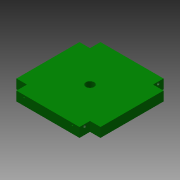
# Autodesk Inventor part: PEEKplate
Saved by Autodesk Inventor 2015 SP1 (Build 190203100, 203)
## iProperties
Created: 2015-09-28
Part Number: PEEKplate
Material: Generic
Document SubType Name: Modeling
Designer: I Rabey
Density: 1 g/cm^3
Appearance: Default
Author: I Rabey
Autodesk Inventor part; units mm, degrees
ref_plane "YZ Plane" through (0, 0, 0) normal (1, 0, 0) x (0, 1, 0)
ref_plane "XZ Plane" through (0, 0, 0) normal (0, 1, 0) x (-1, 0, 0)
ref_plane "XY Plane" through (0, 0, 0) normal (0, 0, 1) x (1, 0, 0)
sketch "Sketch1" plane through (0, 0, 0) normal (0, 1, 0) x (-1, 0, 0)
  line L0 (51.3, 38.5) -> (51.3, -38.5)
  line L1 (51.3, -38.5) -> (38.5, -38.5)
  line L2 (38.5, -38.5) -> (38.5, -51.3)
  line L3 (38.5, -51.3) -> (-38.5, -51.3)
  line L4 (-38.5, -51.3) -> (-38.5, -38.5)
  line L5 (-38.5, -38.5) -> (-51.3, -38.5)
  line L6 (-51.3, -38.5) -> (-51.3, 38.5)
  line L7 (-51.3, 38.5) -> (-38.5, 38.5)
  line L8 (-38.5, 38.5) -> (-38.5, 51.3)
  line L9 (-38.5, 51.3) -> (38.5, 51.3)
  line L10 (38.5, 51.3) -> (38.5, 38.5)
  line L11 (38.5, 38.5) -> (51.3, 38.5)
  circle A0 centre (0, 0) radius 5
  dimension "d0" = 77
  dimension "d1" = 12.8
  dimension "d2" = 12.8
  dimension "d3" = 77
  dimension "d4" = 12.8
  dimension "d5" = 12.8
  dimension "d6" = 77
  dimension "d7" = 12.8
  dimension "d8" = 12.8
  dimension "d9" = 77
  dimension "d10" = 12.8
  dimension "d11" = 12.8
  dimension "d12" = 38.5
  dimension "d13" = 51.3
  dimension "d14" = 10
  constraints: 24 end point, 7 point on line, 3 perpendicular, 1 centre point, 1 coincident, 1 horizontal, 1 vertical
  measures "d0" distance of L0.start L0.end
  measures "d1" distance of L0.end L1.end
  measures "d2" distance of L1.end L2.end
  measures "d3" distance of L2.end L3.end
  measures "d4" distance of L3.end L4.end
  measures "d5" distance of L4.end L5.end
  measures "d6" distance of L5.end L6.end
  measures "d7" distance of L6.end L7.end
  measures "d8" distance of L7.end L8.end
  measures "d9" distance of L8.end L9.end
  measures "d10" distance of L9.end L10.end
  measures "d11" distance of L10.end L11.end
  measures "d12" distance from line of L1 point (0, 0)
  measures "d13" distance from line of L0 point (0, 0)
  measures "d14" diameter of A0
extrude "Extrusion1" add sketch "Sketch1" along normal blind 11.5
sketch "Sketch2" plane through (38.5, 0, 51.3) normal (1, 0, 0) x (0, 0, -1)
  circle A0 centre (6.4, 9) radius 1.65
  line L0 (0, 0) -> (0, 11.5) projected
  line L1 (0, 11.5) -> (12.8, 11.5) projected
  point P0 (51.3, 0)
  dimension "d17" = 3.3
  dimension "d18" = 6.4
  dimension "d19" = 2.5
  constraints: 1 centre point
  measures "d17" diameter of A0
  measures "d18" distance from line of A0.centre L0
  measures "d19" distance from line of L1 A0.centre
hole "Hole1" at (38.5, 9, 44.9) direction (-1, 0, 0) diameter 3.3 depth 10 tip angle 118
thread "Thread1" size "M3.5x0.6" class "6H" standard "ANSI Metric M Profile" full length
sketch "Sketch3" plane through (-38.5, 0, 51.3) normal (0, 0, 1) x (1, 0, 0)
  circle A0 centre (68, 9) radius 0.5
  line L0 (0, 11.5) -> (77, 11.5) projected
  line L1 (77, 0) -> (77, 11.5) projected
  point P0 (38.5, 0)
  dimension "d29" = 1
  dimension "d30" = 2.5
  dimension "d31" = 9
  constraints: 1 centre point
  measures "d29" diameter of A0
  measures "d30" distance from line of L0 A0.centre
  measures "d31" distance from line of A0.centre L1
hole "Hole2" at (29.5, 9, 51.3) direction (0, 0, -1) diameter 2 depth 5 tip angle 118
sketch "Sketch4" plane through (-38.5, 0, 38.5) normal (-1, 0, 0) x (0, 0, 1)
  circle A0 centre (6.4, 9) radius 1.65
  line L0 (0, 11.5) -> (12.8, 11.5) projected
  line L1 (12.8, 0) -> (12.8, 11.5) projected
  point P0 (-38.5, 0)
  dimension "d39" = 3.3
  dimension "d40" = 2.5
  dimension "d41" = 6.4
  constraints: 1 centre point
  measures "d39" diameter of A0
  measures "d40" distance from line of L0 A0.centre
  measures "d41" distance from line of L1 A0.centre
hole "Hole3" at (-38.5, 9, 44.9) direction (1, 0, 0) diameter 3.3 depth 10 tip angle 118
thread "Thread2" size "M3.5x0.6" class "6H" standard "ANSI Metric M Profile" full length
sketch "Sketch5" plane through (-38.5, 0, 51.3) normal (0, 0, 1) x (1, 0, 0)
  circle A0 centre (9, 9) radius 1
  line L0 (0, 0) -> (0, 11.5) projected
  line L1 (0, 11.5) -> (77, 11.5) projected
  point P0 (38.5, 0)
  dimension "d51" = 2
  dimension "d52" = 9
  dimension "d53" = 2.5
  constraints: 1 centre point
  measures "d51" diameter of A0
  measures "d52" distance from line of A0.centre L0
  measures "d53" distance from line of L1 A0.centre
hole "Hole4" at (-29.5, 9, 51.3) direction (0, 0, -1) diameter 2 depth 5 tip angle 118
sketch "Sketch6" plane through (38.5, 0, -38.5) normal (1, 0, 0) x (0, 0, -1)
  circle A0 centre (6.4, 9) radius 1.65
  line L0 (0, 11.5) -> (12.8, 11.5) projected
  line L1 (12.8, 0) -> (12.8, 11.5) projected
  point P0 (-38.5, 0)
  dimension "d61" = 3.3
  dimension "d62" = 2.5
  dimension "d63" = 6.4
  constraints: 1 centre point
  measures "d61" diameter of A0
  measures "d62" distance from line of A0.centre L0
  measures "d63" distance from line of L1 A0.centre
hole "Hole5" at (38.5, 9, -44.9) direction (-1, 0, 0) diameter 3.3 depth 10 tip angle 118
thread "Thread3" size "M3.5x0.6" class "6H" standard "ANSI Metric M Profile" full length
sketch "Sketch7" plane through (38.5, 0, -51.3) normal (0, 0, -1) x (-1, 0, 0)
  circle A0 centre (9, 9) radius 1
  line L0 (0, 0) -> (0, 11.5) projected
  line L1 (0, 11.5) -> (77, 11.5) projected
  point P0 (38.5, 0)
  dimension "d73" = 2
  dimension "d74" = 9
  dimension "d75" = 2.5
  constraints: 1 centre point
  measures "d73" diameter of A0
  measures "d74" distance from line of L0 A0.centre
  measures "d75" distance from line of L1 A0.centre
hole "Hole6" at (29.5, 9, -51.3) direction (0, 0, 1) diameter 2 depth 5 tip angle 118
sketch "Sketch8" plane through (-38.5, 0, -51.3) normal (-1, 0, 0) x (0, 0, 1)
  circle A0 centre (6.4, 9) radius 1.65
  line L0 (0, 11.5) -> (12.8, 11.5) projected
  line L1 (0, 0) -> (0, 11.5) projected
  point P0 (51.3, 0)
  dimension "d83" = 3.3
  dimension "d84" = 2.5
  dimension "d85" = 6.4
  constraints: 1 centre point
  measures "d83" diameter of A0
  measures "d84" distance from line of L0 A0.centre
  measures "d85" distance from line of L1 A0.centre
hole "Hole7" at (-38.5, 9, -44.9) direction (1, 0, 0) diameter 3.3 depth 10 tip angle 118
thread "Thread4" size "M3.5x0.6" class "6H" standard "ANSI Metric M Profile" full length
sketch "Sketch9" plane through (38.5, 0, -51.3) normal (0, 0, -1) x (-1, 0, 0)
  circle A0 centre (68, 9) radius 1
  line L0 (0, 11.5) -> (77, 11.5) projected
  line L1 (77, 0) -> (77, 11.5) projected
  point P0 (38.5, 0)
  dimension "d95" = 2
  dimension "d96" = 2.5
  dimension "d97" = 9
  constraints: 1 centre point
  measures "d95" diameter of A0
  measures "d96" distance from line of A0.centre L0
  measures "d97" distance from line of L1 A0.centre
hole "Hole8" at (-29.5, 9, -51.3) direction (0, 0, 1) diameter 2 depth 5 tip angle 118
body "Solid1"
